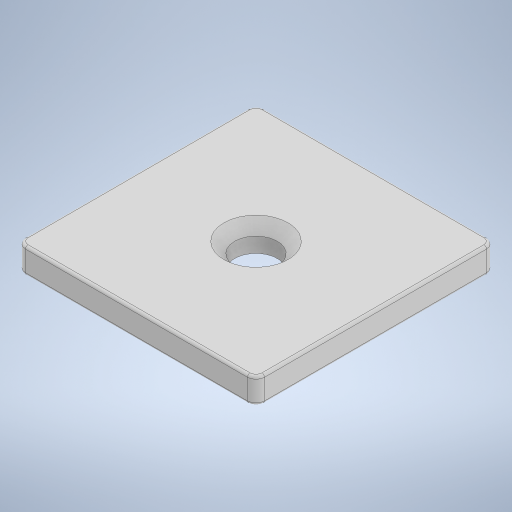
# Autodesk Inventor part: clampPlate
Saved by Autodesk Inventor 2024.2 (Build 282272000, 272)
## iProperties
Created: 2024-05-25
Part Number: clampPlate
Material: Generic
Document SubType Name: Modeling
Designer: user
Density: 1 g/cm^3
Appearance: Default
Author: user
Autodesk Inventor part; units mm, degrees
ref_plane "YZ Plane" through (0, 0, 0) normal (1, 0, 0) x (0, 1, 0)
ref_plane "XZ Plane" through (0, 0, 0) normal (0, 1, 0) x (-1, 0, 0)
ref_plane "XY Plane" through (0, 0, 0) normal (0, 0, 1) x (1, 0, 0)
sketch "Sketch1" plane through (0, 0, 0) normal (0, 1, 0) x (-1, 0, 0)
  line L0 (-14, -14) -> (14, -14)
  line L1 (14, -14) -> (14, 14)
  line L2 (14, 14) -> (-14, 14)
  line L3 (-14, 14) -> (-14, -14)
  line L4 (-14, -14) -> (14, 14) construction
  line L5 (14, -14) -> (-14, 14) construction
  point P0 (0, 0)
  dimension "d0" = 28
  dimension "d1" = 28
  constraints: 12 end point, 2 midpoint, 2 parallel, 1 horizontal, 1 perpendicular
  measures "d0" distance of L2.end L1.end
  measures "d1" distance of L1.end L0.end
extrude "Extrusion1" add sketch "Sketch1" against normal blind 3
hole "Hole1" at (0, 0, 0) direction (0, -1, 0) diameter 5 end through all countersink diameter 7.5 countersink angle 90
fillet "Fillet1" radius 1 4 edges at (14, -1.5, 14) (14, -1.5, -14) (-14, -1.5, -14) (-14, -1.5, 14)
fillet "Fillet2" radius 0.3 16 edges at (13.7071, 0, 13.7071) (14, 0, 0) (13.7071, 0, -13.7071) (0, 0, -14) (-13.7071, 0, -13.7071) (-14, 0, 0) (-13.7071, 0, 13.7071) (0, 0, 14) (-13.7071, -3, 13.7071) (-14, -3, 0) (-13.7071, -3, -13.7071) (0, -3, -14) (13.7071, -3, -13.7071) (14, -3, 0) (13.7071, -3, 13.7071) (0, -3, 14)
body "Solid1"
